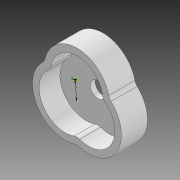
# Autodesk Inventor part: TestHousing
Saved by Autodesk Inventor 2020 (Build 240168000, 168)
## iProperties
Created: 2021-05-17
Part Number: TestHousing
Material: Generic
Document SubType Name: Modeling
Designer: DDeGo
Density: 1 g/cm^3
Appearance: Default
Author: DDeGo
Autodesk Inventor part; units mm, degrees
ref_plane "YZ Plane" through (0, 0, 0) normal (1, 0, 0) x (0, 1, 0)
ref_plane "XZ Plane" through (0, 0, 0) normal (0, 1, 0) x (-1, 0, 0)
ref_plane "XY Plane" through (0, 0, 0) normal (0, 0, 1) x (1, 0, 0)
sketch "Sketch1" plane through (0, 0, 0) normal (0, 0, 1) x (1, 0, 0)
  circle A0 centre (0, 3.8477) radius 10 construction
  line L0 (0, 0) -> (0, 3.8477) construction
  circle A1 centre (0, 3.8477) radius 12.5
  circle A2 centre (-3.3322, -1.9238) radius 10 construction
  line L1 (0, 0) -> (-3.3322, -1.9238) construction
  circle A3 centre (-3.3322, -1.9238) radius 12.5
  circle A4 centre (3.3322, -1.9238) radius 10 construction
  line L2 (0, 0) -> (3.3322, -1.9238) construction
  circle A5 centre (3.3322, -1.9238) radius 12.5
  line L3 (11.9924, -6.9238) -> (-9.8314, 5.6762) construction
  point P0 (12.0997, 6.9858)
  point P1 (-12.0997, 6.9858)
  point P2 (0, -13.9715)
  dimension "d1" = 20
  dimension "d2" = 2.5
  dimension "d5" = 360
  dimension "d19" = 6.6644
  dimension "d20" = 25.2
  constraints: 8 end point, 5 coincident, 3 centre point, 1 point on line, 1 vertical, 26 other
  measures "d19" distance of L0.end L2.end
  measures "d20" distance of L3.start L3.end
extrude "Extrusion1" add sketch "Sketch1" along normal blind 10
sketch "Sketch2" plane through (0, 0, 10) normal (0, 0, 1) x (1, 0, 0)
  arc A0 (12.0997, 6.9858) -> (-12.0997, 6.9858) centre (0, 3.8477) ccw projected
  circle A1 centre (0, 3.8477) radius 10
  arc A2 (-12.0997, 6.9858) -> (0, -13.9715) centre (-3.3322, -1.9238) ccw projected
  circle A3 centre (-3.3322, -1.9238) radius 10
  arc A4 (0, -13.9715) -> (12.0997, 6.9858) centre (3.3322, -1.9238) ccw projected
  circle A5 centre (3.3322, -1.9238) radius 10
  point P0 (0, 0)
  point P1 (0, 7.5047)
  point P2 (6.4992, -3.7523)
  point P3 (-6.4992, -3.7523)
  point P4 (9.8314, 5.6762)
  point P5 (-9.8314, 5.6762)
  point P6 (0, -11.3523)
  dimension "d10" = 20
  constraints: 3 centre point, 3 coincident, 2 equal radius
  measures "d10" diameter of A3
extrude "Extrusion2" cut sketch "Sketch2" against normal blind 8 contours A1 A3 A5 | A1 A5 A3 | A5 A3 A1 | A3 A5 A1 | A1 A5 A3 | A3 A5 A1 | A1 A5 A3
sketch "Sketch3" plane through (0, 0, 2) normal (0, 0, 1) x (1, 0, 0)
  circle A0 centre (0, 0) radius 3
  dimension "d13" = 6
  constraints: 1 centre point, 1 coincident
  measures "d13" diameter of A0
extrude "Extrusion3" cut sketch "Sketch3" against normal blind 8
fillet "Fillet1" radius 2 6 edges at (-9.8314, 5.6762, 6) (-12.0997, 6.9858, 5) (12.0997, 6.9858, 5) (9.8314, 5.6762, 6) (0, -11.3523, 6) (0, -13.9715, 5)
sketch "Sketch4" plane through (0, 0, 10) normal (0, 0, 1) x (1, 0, 0)
  circle A0 centre (-0.6635, 6.9685) radius 0.5
  point P0 (0, 0)
  dimension "d17" = 1
  dimension "d18" = 7
  constraints: 1 centre point
  measures "d17" diameter of A0
  measures "d18" distance of A0.centre point (0, 0)
body "Solid1"
